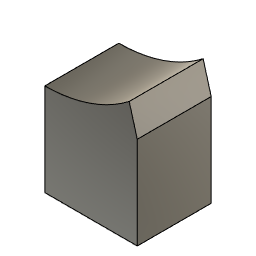
switch v2 (Autodesk Fusion 360 design; units mm, degrees)
Autodesk Fusion 360 part; units mm, degrees
sketch "Sketch1" plane through (0, 0, 0) normal (0, 1, 0) x (1, 0, 0)
  line L0 (0, 0) -> (10, 0)
  line L1 (10, 0) -> (10, -10)
  line L2 (0, -10) -> (0, 0)
  line L3 (10, -10) -> (9.131, -13.1109)
  arc A0 (9.131, -13.1109) -> (0, -10) centre (0, -24.956) ccw
  dimension "d1" = 10
  dimension "d2" = 10
  dimension "d3" = 3.23
  constraint horizontal L0
  constraint vertical L1
  constraint vertical L2
  constraint coincident L0.start L2.end
  measures "d1" distance of L0.start L0.end
  measures "d2" distance of L0.start L2.start
  measures "d3" distance of L1.end L3.end
extrude "Extrude1" add sketch "Sketch1" along normal blind 8
